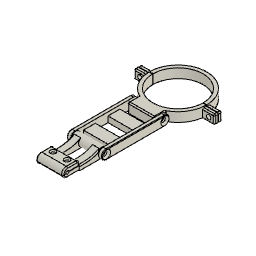
スポンジ受け v0 (Autodesk Fusion 360 design; units mm, degrees)
Autodesk Fusion 360 part; units mm, degrees
note: some values were not read from the file. Set by a fixed rule: which face or edge a step refers to.
sketch "スケッチ1" plane through (0, 0, 0) normal (0, 0, 1) x (1, 0, 0)
  circle A0 centre (0, 50) radius 21.5
  circle A1 centre (0, 50) radius 24.5
  line L0 (0, 50) -> (30, 50)
  line L1 (0, 50) -> (-30, 50)
  dimension "d1" = 43
  dimension "d2" = 49
  constraint concentric A0 A1
  constraint coincident A0.centre A1.centre
  constraint horizontal L0
  constraint parallel L0 L1
  measures "d1" diameter of A0
  measures "d2" diameter of A1
extrude "押し出し1" add sketch "スケッチ1" along normal blind 8 contours A0 A1 L0 L1 picked at (-17.9877, 65.0298) makes body 1
move_face "面を移動1" by (0, 0.2, 0) 2 faces at (-22.5, 50, 5.3333) (22.5, 50, 5.3333) on bodies 1
sketch "スケッチ2" plane through (0, 50.2, 0) normal (0, -1, 0) x (1, 0, 0)
  line L0 (21.4991, 0) -> (24.4992, 0)
  line L1 (24.4992, 0) -> (24.4992, 8)
  line L2 (24.4992, 8) -> (21.4991, 8)
  line L3 (21.4991, 8) -> (21.4991, 0)
  line L4 (24.4992, 0) -> (34.4992, 0)
  line L5 (34.4992, 0) -> (34.4992, 7)
  line L6 (34.4992, 7) -> (24.4992, 7)
  circle A0 centre (29.4992, 3.5) radius 1.9
  line L7 (24.4992, 7) -> (22.5, 7)
  line L8 (22.5, 7) -> (22.5, 0)
  line L9 (24.4992, 0) -> (22.5, 0)
  dimension "d5" = 10
  dimension "d6" = 3.8
  constraint horizontal L4
  constraint vertical L5
  constraint horizontal L6
  constraint coincident L0.end L1.start
  constraint coincident L0 L8.end
  constraint perpendicular L0 L8
  constraint perpendicular L8 L9
  measures "d5" distance of L0.end L4.end
  measures "d6" diameter of A0
extrude "押し出し2" add sketch "スケッチ2" against normal blind 3 separate body contours L0 L1 L7 L8 L9 | L1 L4 L5 L6 makes body 2
fillet "フィレット1" radius 1 3 edges at (28.4996, 53.2, 7) (34.4992, 53.2, 3.5) (34.4992, 51.7, 7) on bodies 2
move_face "面を移動2" to x (1, 0, 0) y (0, 1, 0) z (0, 0, 1) at (0, 0, -0.5) 1 faces at (31.3968, 52.2, 3.4053) on bodies 2
sketch "スケッチ3" plane through (0, 53.2, 0) normal (0, 1, 0) x (-1, 0, 0)
  line L0 (-22.5, 6) -> (-33.4992, 6)
  line L1 (-33.4992, 6) -> (-33.4992, 0)
  line L2 (-33.4992, 0) -> (-22.5, 0)
  line L3 (-22.5, 0) -> (-22.5, 6)
  circle A0 centre (-29.4992, 3) radius 1.9
mirror "ミラー1" about plane through (0, 0, 0) normal (1, 0, 0) of bodies 2 makes body 3
combine "結合1" operation add target body 1 tool bodies 3 2
ref_plane "作業平面1" through (15, 50, 0) normal (0, -1, 0) x (1, 0, 0)
mirror "ミラー2" about plane through (15, 50, 0) normal (0, -1, 0) of bodies 1 makes body 4
sketch "スケッチ4" plane through (0, 0, 0) normal (0, 0, 1) x (1, 0, 0)
  line L0 (0, 24) -> (0, 28)
  line L1 (12, 24) -> (12, 1)
  line L2 (12, 1) -> (15, 1)
  line L3 (15, 1) -> (15, 24)
  line L4 (0, 20) -> (0, 24)
  line L5 (11.5, 28.372) -> (0, 26)
  line L6 (12, 24) -> (15, 24)
  line L7 (11.5, 18.372) -> (0, 18.372)
  line L8 (0, 18.372) -> (0, 20)
  line L9 (11.5, 18.372) -> (11.5, 28.372)
  dimension "d19" = 15
  dimension "d22" = 10
  constraint perpendicular L1 L2
  constraint midpoint L0 L5.end
  constraint perpendicular L7 L9
  measures "d19" distance of L0.start L3.end
  measures "d22" distance of L5.start L7.start
extrude "押し出し3" add sketch "スケッチ4" along normal blind 8 separate body contours L0 L4 L5 L7 L8 L9 makes body 5
fillet "フィレット2" radius 1 3 edges at (5.75, 18.372, 8) (11.5, 23.372, 8) (11.5, 18.372, 4) on bodies 5
sketch "スケッチ5" plane through (0, 0, 0) normal (0, 0, 1) x (1, 0, 0)
sketch "スケッチ6" plane through (11.5, 0, 0) normal (1, 0, 0) x (0, 1, 0)
  line L0 (19.372, 7) -> (19.372, 0)
  line L1 (19.372, 0) -> (28.372, 0)
  line L2 (28.372, 0) -> (28.372, 7)
  line L3 (28.372, 7) -> (19.372, 7)
  line L4 (19.372, 7) -> (28.372, 0) construction
  line L5 (28.372, 7) -> (19.372, 0) construction
  circle A0 centre (23.872, 3.5) radius 1.4
  dimension "d27" = 2.8
  constraint coincident L0.start L3.end
  constraint coincident L1.end L2.start
  constraint coincident L2.end L3.start
  constraint coincident L0.end L1.start
  constraint midpoint L4 A0.centre
  measures "d27" diameter of A0
extrude "押し出し4" cut sketch "スケッチ6" against normal blind 16 contours A0 bodies 5
mirror "ミラー3" about plane through (0, 24, 0) normal (-1, 0, 0) of bodies 5 merged
combine "結合2" operation add target body 4 tool bodies 5
sketch "スケッチ7" plane through (0, 0, 0) normal (0, 0, 1) x (1, 0, 0)
  line L0 (17.1897, 26.9527) -> (27.1897, 26.9527)
  line L1 (27.1897, 26.9527) -> (27.1897, -33.0473)
  line L2 (27.1897, -33.0473) -> (17.1897, -33.0473)
  line L3 (17.1897, -33.0473) -> (17.1897, 26.9527)
  dimension "d32" = 10
  dimension "d33" = 60
  constraint horizontal L0
  constraint vertical L1
  constraint horizontal L2
  constraint vertical L3
  measures "d32" distance of L0.start L0.end
  measures "d33" distance of L0.start L2.end
move_face "面を移動3" to x (1, 0, 0) y (0, 1, 0) z (0, 0, 1) at (0, 0, 1) 2 faces at (7.6667, 25.265, 3.3606) (-7.6667, 25.265, 3.3606) on bodies 4
move_face "面を移動4" to x (1, 0, 0) y (0, 1, 0) z (0, 0, 1) at (0, 0, -0.5) 1 faces at (3.8333, 25.265, 4.3606) on bodies 4
move_face "面を移動5" to x (1, 0, 0) y (0, 1, 0) z (0, 0, 1) at (0, 0, 0.5) 1 faces at (3.8333, 25.265, 3.8606) on bodies 4
sketch "スケッチ10" plane through (11.5, 0, 0) normal (1, 0, 0) x (0, 1, 0)
  line L0 (28.3667, 0) -> (28.3667, 7)
  line L1 (28.3667, 7) -> (19.372, 7)
  line L2 (19.372, 7) -> (19.372, 0)
  line L3 (19.372, 0) -> (28.3667, 0)
  circle A0 centre (23.872, 4.5) radius 1.4
  circle A1 centre (23.872, 4.5) radius 4
  circle A2 centre (-26.128, 4.5) radius 4
  circle A3 centre (-26.128, 4.5) radius 1.85
  circle A4 centre (23.872, 4.5) radius 1.85
  line L4 (-26.128, 8.5) -> (23.872, 8.5)
  line L5 (-26.128, 0.5) -> (23.872, 0.5)
  line L6 (-22.128, 4.5) -> (-26.128, 4.5)
  dimension "d49" = 8
  dimension "d50" = 50
  dimension "d51" = 8
  dimension "d52" = 3.7
  dimension "d53" = 3.7
  constraint concentric A0 A1
  constraint coincident A2.centre A3.centre
  constraint concentric A0 A4
  constraint coincident A2 L4.start
  constraint coincident A1 L4.end
  constraint tangent A1 L4
  constraint coincident A2 L6.start
  measures "d49" diameter of A1
  measures "d50" distance of A0.centre A2.centre
  measures "d51" diameter of A2
  measures "d52" diameter of A3
  measures "d53" diameter of A4
extrude "押し出し5" add sketch "スケッチ10" along normal blind 3 separate body contours L1 A1 | L1 A1 | L1 L2 A1 A2 L4 L5 | L1 L2 A1 L5 | A2 makes body 6
chamfer "面取り1" distance 1.6 angle 45 1 edges at (14.5, 22.1471, 5.169) on bodies 6
chamfer "面取り2" distance 1.6 angle 45 1 edges at (14.5, -27.8529, 5.169) on bodies 6
move_body "移動1" bodies 6 to x (1, 0, 0) y (0, 1, 0) z (0, 0, 1) at (0.5, 0, 0)
mirror "ミラー4" about plane through (0, 0, 0) normal (1, 0, 0) of bodies 6 makes body 7
sketch "スケッチ11" plane through (12, 0, 0) normal (-1, 0, 0) x (0, -1, 0)
  circle A0 centre (-23.872, 4.5) radius 1.85
  circle A1 centre (26.128, 4.5) radius 1.85
  arc A2 (26.128, 0.5) -> (26.128, 8.5) centre (26.128, 4.5) ccw
  line L0 (26.128, 8.5) -> (-23.872, 8.5)
  arc A3 (-23.872, 8.5) -> (-23.872, 0.5) centre (-23.872, 4.5) ccw
  line L1 (-23.872, 0.5) -> (26.128, 0.5)
  line L2 (-12.2235, 0.5) -> (-2.0804, 0.5)
  line L3 (-2.0804, 5.5) -> (-12.2235, 5.5)
  line L4 (-12.2235, 5.5) -> (-12.2235, 0.5)
  line L5 (-2.0804, 0.5) -> (-2.0804, 5.5)
  line L6 (8.7765, 5.5) -> (8.7765, 0.5)
  line L7 (8.7765, 0.5) -> (18.9196, 0.5)
  line L8 (18.9196, 0.5) -> (18.9196, 5.5)
  line L9 (18.9196, 5.5) -> (8.7765, 5.5)
  dimension "d64" = 5
  dimension "d65" = 5
  constraint horizontal L2
  constraint horizontal L3
  constraint vertical L4
  constraint coincident L1 L2.start
  constraint coincident L1 L2.end
  constraint perpendicular L3 L5
  constraint horizontal L7
  constraint horizontal L9
  constraint vertical L6
  constraint perpendicular L8 L9
  measures "d64" distance of L2.start L3.end
  measures "d65" distance of L6.end L6.start
extrude "押し出し6" add sketch "スケッチ11" along normal blind 25 contours L1 L6 L7 L8 L9 | L1 L2 L3 L4 L5 bodies 7 6
fillet "フィレット3" radius 0.5 8 edges at (15, -1.128, 0.5) (15, 27.872, 4.5) (15, -1.128, 8.5) (15, -30.128, 4.5) (-15, -1.128, 0.5) (-15, 27.872, 4.5) (-15, -1.128, 8.5) (-15, -30.128, 4.5) on bodies 7
sketch "スケッチ12" plane through (-12, 0, 0) normal (1, 0, 0) x (0, 1, 0)
  line L0 (-8.7765, 5.5) -> (-8.7765, 0.5)
  line L1 (-8.7765, 0.5) -> (2.0804, 0.5)
  line L2 (2.0804, 0.5) -> (2.0804, 5.5)
  line L3 (2.0804, 5.5) -> (12.2235, 5.5)
  line L4 (12.2235, 5.5) -> (12.2235, 0.5)
  line L5 (12.2235, 0.5) -> (23.872, 0.5)
  arc A0 (23.872, 0.5) -> (23.872, 8.5) centre (23.872, 4.5) ccw
  line L6 (23.872, 8.5) -> (-26.128, 8.5)
  arc A1 (-26.128, 8.5) -> (-26.128, 0.5) centre (-26.128, 4.5) ccw
  line L7 (-26.128, 0.5) -> (-18.9196, 0.5)
  line L8 (-18.9196, 0.5) -> (-18.9196, 5.5)
  line L9 (-18.9196, 5.5) -> (-8.7765, 5.5)
  circle A2 centre (-26.128, 4.5) radius 1.85
  circle A3 centre (23.872, 4.5) radius 1.85
  circle A4 centre (-26.128, 4.5) radius 4
  dimension "d70" = 8
  constraint concentric A1 A4
  measures "d70" diameter of A4
extrude "押し出し7" add sketch "スケッチ12" along normal blind 12 separate body contours A1 A4 | A2 makes body 8
move_face "面を移動6" by (0.5, 0, 0) 1 faces at (-12, -27.4081, 4.6898) on bodies 8
sketch "スケッチ13" plane through (-11.5, 0, 0) normal (-1, 0, 0) x (0, -1, 0)
  circle A0 centre (26.128, 4.5) radius 4
  line L0 (26.128, 0.5) -> (56.128, 0.5)
  line L1 (46, 3.5) -> (46, 0.5)
  line L2 (46, 8.5) -> (46, 3.5)
  circle A1 centre (56.128, 4.5) radius 1.25
  line L3 (56.128, 8.5) -> (26.128, 8.5)
  line L4 (54.878, 4.5) -> (46, 4.5)
  line L5 (57.3228, 4.1323) -> (59.9511, 3.3235)
  arc A2 (52.128, 4.5) -> (56.128, 8.5) centre (56.128, 4.5) ccw
  dimension "d76" = 30
  dimension "d79" = 8
  dimension "d80" = 2.5
  constraint coincident A0 L0.start
  constraint horizontal L0
  constraint coincident L0 L1.end
  constraint perpendicular L0 L1
  constraint coincident L0.end A2
  constraint concentric A1 A2
  constraint coincident A0 L3.end
  constraint tangent A0 L3
  constraint coincident L3 L2.start
  constraint coincident L2 L4.end
  constraint perpendicular L2 L4
  constraint coincident L5.end A2
  constraint coincident A1 L5.start
  constraint coincident A1 L4.start
  constraint coincident L4 A2.start
  measures "d76" distance of L0.start L0.end
  measures "d79" diameter of A2
  measures "d80" diameter of A1
extrude "押し出し8" add sketch "スケッチ13" against normal blind 11.5 separate body contours L0 L1 L2 L4 A2 | A1 L4 L5 A2 makes body 9
extrude "押し出し9" add sketch "スケッチ13" against normal blind 11.5 separate body contours L2 A1 L3 L4 L5 A2 makes body 10
mirror "ミラー5" about plane through (0, 0, 0) normal (1, 0, 0) of bodies 8 merged
sketch "スケッチ14" plane through (0, 0, 8.5) normal (0, 0, 1) x (-1, 0, 0)
  line L0 (11.5, 46) -> (11.5, 56.128)
  line L1 (11.5, 56.128) -> (0, 56.128)
  line L2 (0, 56.128) -> (0, 46)
  line L3 (0, 46) -> (11.5, 46)
  circle A0 centre (6, 51) radius 1.35
  circle A1 centre (6, 51) radius 0.8
  dimension "d87" = 2.7
  dimension "d91" = 1.6
  constraint concentric A0 A1
  measures "d87" diameter of A0
  measures "d91" diameter of A1
extrude "押し出し10" cut sketch "スケッチ14" against normal blind 11 contours A0 | A1 bodies 10
chamfer "面取り3" distance 1 angle 45 1 edges at (-4.7414, -51.4882, 8.5) on bodies 10
extrude "押し出し11" cut sketch "スケッチ14" against normal blind 10 contours A1 bodies 9
move_face "面を移動7" by (0, 0, 0.3) 1 faces at (-1.555, -50.5589, 4.5) on bodies 10
move_face "面を移動8" by (0, -0.0882, 0.2867) 1 faces at (-7.6667, -58.1989, 3.8627) on bodies 10
mirror "ミラー6" about plane through (0, 0, 0) normal (1, 0, 0) of bodies 9 10 merged
sketch "スケッチ15" plane through (0, 0, 0) normal (1, 0, 0) x (0, 1, 0)
  circle A0 centre (-26.128, 4.5) radius 4
  line L0 (-46, 0.5) -> (-26.128, 0.5)
  spline S0 degree 5 poles (-46, 4.5) (-45.6231, 4.4988) (-44.8655, 4.4995) (-43.7177, 4.5101) (-42.1706, 4.5445) (-40.2413, 4.6295) (-38.3548, 4.77) (-36.5432, 4.9833) (-34.8216, 5.2898) (-33.1713, 5.7106) (-31.5528, 6.2669) (-30.2469, 6.837) (-29.2437, 7.3425) (-28.5619, 7.7154) (-28.2178, 7.9107) knots 0 0 0 0 0 0 0.1 0.2 0.3 0.4 0.5 0.6 0.7 0.8 0.9 1 1 1 1 1 1
  line L1 (-47.9168, 4.5063) -> (-44.0832, 4.4937)
  line L2 (-30.0723, 6.858) -> (-26.3634, 8.9634)
  line L3 (-46, 4.5) -> (-46, 0.5)
  point P0 (-26.128, 0.5)
  point P1 (-46, 0.5)
  point P2 (-46, 4.5)
  point P3 (-36.3352, 5.0416)
  constraint coincident P1 L0.start
  constraint coincident P0 L0.end
  constraint coincident P2 S0.start
  constraint coincident A0 S0.end
  constraint midpoint P2 L1
  constraint midpoint S0.end L2
extrude "押し出し12" add sketch "スケッチ15" along normal blind -5 and the other way blind 11.5 separate body contours A0 L0 S0 L3 makes body 11
mirror "ミラー7" about plane through (0, 0, 0) normal (1, 0, 0) of bodies 11 makes body 12
combine "結合3" operation add target body 12 tool bodies 8 11
fillet "フィレット4" radius 2 1 edges at (0, -46, 8.5) on bodies 10
fillet "フィレット5" radius 1 8 edges at (-11.5, -59.2542, 6.9954) (-11.5, -52.064, 8.5) (-11.5, -46.5858, 7.9142) (-11.5, -46, 5.65) (11.5, -59.2542, 6.9954) (11.5, -52.064, 8.5) (11.5, -46.5858, 7.9142) (11.5, -46, 5.65) on bodies 10
fillet "フィレット6" radius 1 2 edges at (11.5, -51.064, 0.5) (11.5, -58.5044, 1.2824) on bodies 9
fillet "フィレット7" radius 1 2 edges at (-11.5, -51.064, 0.5) (-11.5, -58.5044, 1.2824) on bodies 9
fillet "フィレット8" radius 1 2 edges at (11.5, -36.5654, 5.0066) (-11.5, -36.5654, 5.0066) on bodies 12
sketch "スケッチ16" plane through (-11.5, 0, 0) normal (-1, 0, 0) x (0, -1, 0)
  arc A0 (29.8601, 5.9394) -> (26.128, 0.5) centre (26.128, 4.5) ccw
  line L0 (26.128, 0.5) -> (46, 0.5)
  line L1 (46, 0.5) -> (46, 3.5)
  spline S0 degree 3 poles (29.8601, 5.9394) (30.5342, 5.6282) (31.2224, 5.3468) (33.3808, 4.5903) (34.8926, 4.2434) (36.4189, 4.0174) (38.003, 3.7828) (39.6022, 3.6647) (42.7998, 3.5201) (44.3997, 3.4948) (46, 3.5) knots -1.646275 -1.646275 -1.646275 -1.646275 -1.423697 -1.423697 -0.960811 -0.960811 -0.960811 -0.480406 -0.480406 -0.000327 -0.000327 -0.000327 -0.000327
  circle A1 centre (26.128, 4.5) radius 1.4
  dimension "d115" = 2.8
  constraint concentric A0 A1
  measures "d115" diameter of A1
extrude "押し出し13" cut sketch "スケッチ16" against normal blind 32 contours A1 bodies 12
